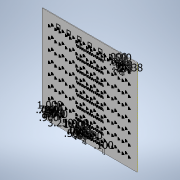
# Autodesk Inventor part: Cube_Pcb
Saved by Autodesk Inventor 2020 (Build 240168000, 168)
## iProperties
Created: 2019-12-01
Part Number: Cube_Pcb
Material: Generic
Document SubType Name: Modeling
Designer: torto
Density: 1 g/cm^3
Appearance: Default
Author: torto
Autodesk Inventor part; units mm, degrees
(part 1 of 2)
ref_plane "YZ Plane" through (0, 0, 0) normal (1, 0, 0) x (0, 1, 0)
ref_plane "XZ Plane" through (0, 0, 0) normal (0, 1, 0) x (-1, 0, 0)
ref_plane "XY Plane" through (0, 0, 0) normal (0, 0, 1) x (1, 0, 0)
sketch "Sketch1" plane through (0, 0, 0) normal (0, 0, 1) x (1, 0, 0)
  line L0 (0, 0) -> (228.6, 0)
  line L1 (228.6, 0) -> (228.6, 228.6)
  line L2 (228.6, 228.6) -> (0, 228.6)
  line L3 (0, 228.6) -> (0, 0)
  dimension "d0" = 228.6
  dimension "d1" = 228.6
  constraints: 8 end point, 2 parallel, 1 horizontal, 1 perpendicular
  measures "d0" distance of L2.end L1.end
  measures "d1" distance of L1.end L0.end
extrude "Extrusion1" add sketch "Sketch1" along normal blind 1.524
sketch "Details" plane through (0, 0, 1.524) normal (0, 0, 1) x (1, 0, 0)
  line L0 (0, 0) -> (82.55, 0) construction
  line L1 (82.55, 0) -> (82.55, 12.7) construction
  line L2 (82.55, 12.7) -> (0, 12.7) construction
  line L3 (0, 12.7) -> (0, 0) construction
  line L4 (82.55, 12.7) -> (146.05, 12.7)
  line L5 (146.05, 12.7) -> (146.05, 15.24)
  line L6 (146.05, 15.24) -> (82.55, 15.24)
  line L7 (82.55, 15.24) -> (82.55, 12.7)
  line L8 (82.55, 12.7) -> (100.33, 12.7)
  line L9 (100.33, 12.7) -> (100.33, 15.24)
  line L10 (100.33, 15.24) -> (82.55, 15.24)
  line L11 (82.55, 15.24) -> (82.55, 12.7)
  line L12 (105.41, 15.24) -> (105.41, 12.7)
  line L13 (123.19, 12.7) -> (123.19, 15.24)
  line L14 (128.27, 15.24) -> (128.27, 12.7)
  line L15 (146.05, 12.7) -> (146.05, 15.24)
  line L16 (82.55, 40.64) -> (82.55, 38.1)
  line L17 (82.55, 38.1) -> (100.33, 38.1)
  line L18 (100.33, 38.1) -> (100.33, 40.64)
  line L19 (100.33, 40.64) -> (82.55, 40.64)
  line L20 (146.05, 40.64) -> (82.55, 40.64)
  line L21 (105.41, 40.64) -> (105.41, 38.1)
  line L22 (82.55, 38.1) -> (146.05, 38.1)
  line L23 (146.05, 38.1) -> (146.05, 40.64)
  line L24 (128.27, 40.64) -> (128.27, 38.1)
  line L25 (123.19, 38.1) -> (123.19, 40.64)
  line L26 (82.55, 66.04) -> (82.55, 63.5)
  line L27 (82.55, 63.5) -> (100.33, 63.5)
  line L28 (100.33, 63.5) -> (100.33, 66.04)
  line L29 (100.33, 66.04) -> (82.55, 66.04)
  line L30 (146.05, 66.04) -> (82.55, 66.04)
  line L31 (105.41, 66.04) -> (105.41, 63.5)
  line L32 (82.55, 63.5) -> (146.05, 63.5)
  line L33 (146.05, 63.5) -> (146.05, 66.04)
  line L34 (128.27, 66.04) -> (128.27, 63.5)
  line L35 (123.19, 63.5) -> (123.19, 66.04)
  line L36 (82.55, 91.44) -> (82.55, 88.9)
  line L37 (82.55, 88.9) -> (100.33, 88.9)
  line L38 (100.33, 88.9) -> (100.33, 91.44)
  line L39 (100.33, 91.44) -> (82.55, 91.44)
  line L40 (146.05, 91.44) -> (82.55, 91.44)
  line L41 (105.41, 91.44) -> (105.41, 88.9)
  line L42 (82.55, 88.9) -> (146.05, 88.9)
  line L43 (146.05, 88.9) -> (146.05, 91.44)
  line L44 (128.27, 91.44) -> (128.27, 88.9)
  line L45 (123.19, 88.9) -> (123.19, 91.44)
  line L46 (82.55, 116.84) -> (82.55, 114.3)
  line L47 (82.55, 114.3) -> (100.33, 114.3)
  line L48 (100.33, 114.3) -> (100.33, 116.84)
  line L49 (100.33, 116.84) -> (82.55, 116.84)
  line L50 (146.05, 116.84) -> (82.55, 116.84)
  line L51 (105.41, 116.84) -> (105.41, 114.3)
  line L52 (82.55, 114.3) -> (146.05, 114.3)
  line L53 (146.05, 114.3) -> (146.05, 116.84)
  line L54 (128.27, 116.84) -> (128.27, 114.3)
  line L55 (123.19, 114.3) -> (123.19, 116.84)
  line L56 (82.55, 142.24) -> (82.55, 139.7)
  line L57 (82.55, 139.7) -> (100.33, 139.7)
  line L58 (100.33, 139.7) -> (100.33, 142.24)
  line L59 (100.33, 142.24) -> (82.55, 142.24)
  line L60 (146.05, 142.24) -> (82.55, 142.24)
  line L61 (105.41, 142.24) -> (105.41, 139.7)
  line L62 (82.55, 139.7) -> (146.05, 139.7)
  line L63 (146.05, 139.7) -> (146.05, 142.24)
  line L64 (128.27, 142.24) -> (128.27, 139.7)
  line L65 (123.19, 139.7) -> (123.19, 142.24)
  line L66 (82.55, 167.64) -> (82.55, 165.1)
  line L67 (82.55, 165.1) -> (100.33, 165.1)
  line L68 (100.33, 165.1) -> (100.33, 167.64)
  line L69 (100.33, 167.64) -> (82.55, 167.64)
  line L70 (146.05, 167.64) -> (82.55, 167.64)
  line L71 (105.41, 167.64) -> (105.41, 165.1)
  line L72 (82.55, 165.1) -> (146.05, 165.1)
  line L73 (146.05, 165.1) -> (146.05, 167.64)
  line L74 (128.27, 167.64) -> (128.27, 165.1)
  line L75 (123.19, 165.1) -> (123.19, 167.64)
  line L76 (82.55, 193.04) -> (82.55, 190.5)
  line L77 (82.55, 190.5) -> (100.33, 190.5)
  line L78 (100.33, 190.5) -> (100.33, 193.04)
  line L79 (100.33, 193.04) -> (82.55, 193.04)
  line L80 (146.05, 193.04) -> (82.55, 193.04)
  line L81 (105.41, 193.04) -> (105.41, 190.5)
  line L82 (82.55, 190.5) -> (146.05, 190.5)
  line L83 (146.05, 190.5) -> (146.05, 193.04)
  line L84 (128.27, 193.04) -> (128.27, 190.5)
  line L85 (123.19, 190.5) -> (123.19, 193.04)
  line L86 (82.55, 15.24) -> (83.185, 15.24) construction
  line L87 (83.185, 15.24) -> (83.185, 14.478) construction
  line L88 (83.185, 14.478) -> (82.55, 14.478) construction
  line L89 (82.55, 14.478) -> (82.55, 15.24) construction
  line L90 (83.185, 14.478) -> (81.915, 14.478)
  line L91 (81.915, 14.478) -> (81.915, 16.764)
  line L92 (81.915, 16.764) -> (83.185, 16.764)
  line L93 (83.185, 16.764) -> (83.185, 14.478)
  line L94 (86.995, 14.478) -> (86.995, 16.764)
  line L95 (86.995, 16.764) -> (88.265, 16.764)
  line L96 (88.265, 16.764) -> (88.265, 14.478)
  line L97 (88.265, 14.478) -> (86.995, 14.478)
  line L98 (92.075, 14.478) -> (92.075, 16.764)
  line L99 (92.075, 16.764) -> (93.345, 16.764)
  line L100 (93.345, 16.764) -> (93.345, 14.478)
  line L101 (93.345, 14.478) -> (92.075, 14.478)
  line L102 (97.155, 14.478) -> (97.155, 16.764)
  line L103 (97.155, 16.764) -> (98.425, 16.764)
  line L104 (98.425, 16.764) -> (98.425, 14.478)
  line L105 (98.425, 14.478) -> (97.155, 14.478)
  line L106 (100.33, 12.7) -> (99.695, 12.7) construction
  line L107 (99.695, 12.7) -> (99.695, 13.462) construction
  line L108 (99.695, 13.462) -> (100.33, 13.462) construction
  line L109 (100.33, 13.462) -> (100.33, 12.7) construction
  line L110 (99.695, 13.462) -> (100.9573, 13.462)
  line L111 (100.9573, 13.462) -> (100.9573, 11.176)
  line L112 (100.9573, 11.176) -> (99.695, 11.176)
  line L113 (99.695, 11.176) -> (99.695, 13.462)
  line L114 (94.615, 13.462) -> (95.8773, 13.462)
  line L115 (95.8773, 13.462) -> (95.8773, 11.176)
  line L116 (95.8773, 11.176) -> (94.615, 11.176)
  line L117 (94.615, 11.176) -> (94.615, 13.462)
  line L118 (89.535, 13.462) -> (90.7973, 13.462)
  line L119 (90.7973, 13.462) -> (90.7973, 11.176)
  line L120 (90.7973, 11.176) -> (89.535, 11.176)
  line L121 (89.535, 11.176) -> (89.535, 13.462)
  line L122 (84.455, 13.462) -> (85.7173, 13.462)
  line L123 (85.7173, 13.462) -> (85.7173, 11.176)
  line L124 (85.7173, 11.176) -> (84.455, 11.176)
  line L125 (84.455, 11.176) -> (84.455, 13.462)
  line L126 (81.915, 39.878) -> (81.915, 42.164)
  line L127 (81.915, 42.164) -> (83.185, 42.164)
  line L128 (83.185, 42.164) -> (83.185, 39.878)
  line L129 (83.185, 39.878) -> (81.915, 39.878)
  line L130 (84.455, 38.862) -> (85.7173, 38.862)
  line L131 (85.7173, 38.862) -> (85.7173, 36.576)
  line L132 (85.7173, 36.576) -> (84.455, 36.576)
  line L133 (84.455, 36.576) -> (84.455, 38.862)
  line L134 (88.265, 39.878) -> (86.995, 39.878)
  line L135 (88.265, 42.164) -> (88.265, 39.878)
  line L136 (86.995, 39.878) -> (86.995, 42.164)
  line L137 (86.995, 42.164) -> (88.265, 42.164)
  line L138 (89.535, 36.576) -> (89.535, 38.862)
  line L139 (90.7973, 36.576) -> (89.535, 36.576)
  line L140 (90.7973, 38.862) -> (90.7973, 36.576)
  line L141 (89.535, 38.862) -> (90.7973, 38.862)
  line L142 (92.075, 39.878) -> (92.075, 42.164)
  line L143 (93.345, 39.878) -> (92.075, 39.878)
  line L144 (93.345, 42.164) -> (93.345, 39.878)
  line L145 (92.075, 42.164) -> (93.345, 42.164)
  line L146 (94.615, 36.576) -> (94.615, 38.862)
  line L147 (94.615, 38.862) -> (95.8773, 38.862)
  line L148 (95.8773, 38.862) -> (95.8773, 36.576)
  line L149 (95.8773, 36.576) -> (94.615, 36.576)
  line L150 (97.155, 39.878) -> (97.155, 42.164)
  line L151 (97.155, 42.164) -> (98.425, 42.164)
  line L152 (98.425, 42.164) -> (98.425, 39.878)
  line L153 (98.425, 39.878) -> (97.155, 39.878)
  line L154 (99.695, 38.862) -> (100.9573, 38.862)
  line L155 (100.9573, 38.862) -> (100.9573, 36.576)
  line L156 (100.9573, 36.576) -> (99.695, 36.576)
  line L157 (99.695, 36.576) -> (99.695, 38.862)
  line L158 (81.915, 65.278) -> (81.915, 67.564)
  line L159 (81.915, 67.564) -> (83.185, 67.564)
  line L160 (83.185, 67.564) -> (83.185, 65.278)
  line L161 (83.185, 65.278) -> (81.915, 65.278)
  line L162 (84.455, 64.262) -> (85.7173, 64.262)
  line L163 (85.7173, 64.262) -> (85.7173, 61.976)
  line L164 (85.7173, 61.976) -> (84.455, 61.976)
  line L165 (84.455, 61.976) -> (84.455, 64.262)
  line L166 (88.265, 65.278) -> (86.995, 65.278)
  line L167 (88.265, 67.564) -> (88.265, 65.278)
  line L168 (86.995, 65.278) -> (86.995, 67.564)
  line L169 (86.995, 67.564) -> (88.265, 67.564)
  line L170 (89.535, 61.976) -> (89.535, 64.262)
  line L171 (90.7973, 61.976) -> (89.535, 61.976)
  line L172 (90.7973, 64.262) -> (90.7973, 61.976)
  line L173 (89.535, 64.262) -> (90.7973, 64.262)
  line L174 (92.075, 65.278) -> (92.075, 67.564)
  line L175 (93.345, 65.278) -> (92.075, 65.278)
  line L176 (93.345, 67.564) -> (93.345, 65.278)
  line L177 (92.075, 67.564) -> (93.345, 67.564)
  line L178 (94.615, 61.976) -> (94.615, 64.262)
  line L179 (94.615, 64.262) -> (95.8773, 64.262)
  line L180 (95.8773, 64.262) -> (95.8773, 61.976)
  line L181 (95.8773, 61.976) -> (94.615, 61.976)
  line L182 (97.155, 65.278) -> (97.155, 67.564)
  line L183 (97.155, 67.564) -> (98.425, 67.564)
  line L184 (98.425, 67.564) -> (98.425, 65.278)
  line L185 (98.425, 65.278) -> (97.155, 65.278)
  line L186 (99.695, 64.262) -> (100.9573, 64.262)
  line L187 (100.9573, 64.262) -> (100.9573, 61.976)
  line L188 (100.9573, 61.976) -> (99.695, 61.976)
  line L189 (99.695, 61.976) -> (99.695, 64.262)
  line L190 (81.915, 90.678) -> (81.915, 92.964)
  line L191 (81.915, 92.964) -> (83.185, 92.964)
  line L192 (83.185, 92.964) -> (83.185, 90.678)
  line L193 (83.185, 90.678) -> (81.915, 90.678)
  line L194 (84.455, 89.662) -> (85.7173, 89.662)
  line L195 (85.7173, 89.662) -> (85.7173, 87.376)
  line L196 (85.7173, 87.376) -> (84.455, 87.376)
  line L197 (84.455, 87.376) -> (84.455, 89.662)
  line L198 (88.265, 90.678) -> (86.995, 90.678)
  line L199 (88.265, 92.964) -> (88.265, 90.678)
  line L200 (86.995, 90.678) -> (86.995, 92.964)
  line L201 (86.995, 92.964) -> (88.265, 92.964)
  line L202 (89.535, 87.376) -> (89.535, 89.662)
  line L203 (90.7973, 87.376) -> (89.535, 87.376)
  line L204 (90.7973, 89.662) -> (90.7973, 87.376)
  line L205 (89.535, 89.662) -> (90.7973, 89.662)
  line L206 (92.075, 90.678) -> (92.075, 92.964)
  line L207 (93.345, 90.678) -> (92.075, 90.678)
  line L208 (93.345, 92.964) -> (93.345, 90.678)
  line L209 (92.075, 92.964) -> (93.345, 92.964)
  line L210 (94.615, 87.376) -> (94.615, 89.662)
  line L211 (94.615, 89.662) -> (95.8773, 89.662)
  line L212 (95.8773, 89.662) -> (95.8773, 87.376)
  line L213 (95.8773, 87.376) -> (94.615, 87.376)
  line L214 (97.155, 90.678) -> (97.155, 92.964)
  line L215 (97.155, 92.964) -> (98.425, 92.964)
  line L216 (98.425, 92.964) -> (98.425, 90.678)
  line L217 (98.425, 90.678) -> (97.155, 90.678)
  line L218 (99.695, 89.662) -> (100.9573, 89.662)
  line L219 (100.9573, 89.662) -> (100.9573, 87.376)
  line L220 (100.9573, 87.376) -> (99.695, 87.376)
  line L221 (99.695, 87.376) -> (99.695, 89.662)
  line L222 (81.915, 116.078) -> (81.915, 118.364)
  line L223 (81.915, 118.364) -> (83.185, 118.364)
  line L224 (83.185, 118.364) -> (83.185, 116.078)
  line L225 (83.185, 116.078) -> (81.915, 116.078)
  line L226 (84.455, 115.062) -> (85.7173, 115.062)
  line L227 (85.7173, 115.062) -> (85.7173, 112.776)
  line L228 (85.7173, 112.776) -> (84.455, 112.776)
  line L229 (84.455, 112.776) -> (84.455, 115.062)
  line L230 (88.265, 116.078) -> (86.995, 116.078)
  line L231 (88.265, 118.364) -> (88.265, 116.078)
  line L232 (86.995, 116.078) -> (86.995, 118.364)
  line L233 (86.995, 118.364) -> (88.265, 118.364)
  line L234 (89.535, 112.776) -> (89.535, 115.062)
  line L235 (90.7973, 112.776) -> (89.535, 112.776)
  line L236 (90.7973, 115.062) -> (90.7973, 112.776)
  line L237 (89.535, 115.062) -> (90.7973, 115.062)
  line L238 (92.075, 116.078) -> (92.075, 118.364)
  line L239 (93.345, 116.078) -> (92.075, 116.078)
  line L240 (93.345, 118.364) -> (93.345, 116.078)
  line L241 (92.075, 118.364) -> (93.345, 118.364)
  line L242 (94.615, 112.776) -> (94.615, 115.062)
  line L243 (94.615, 115.062) -> (95.8773, 115.062)
  line L244 (95.8773, 115.062) -> (95.8773, 112.776)
  line L245 (95.8773, 112.776) -> (94.615, 112.776)
  line L246 (97.155, 116.078) -> (97.155, 118.364)
  line L247 (97.155, 118.364) -> (98.425, 118.364)
  line L248 (98.425, 118.364) -> (98.425, 116.078)
  line L249 (98.425, 116.078) -> (97.155, 116.078)
  line L250 (99.695, 115.062) -> (100.9573, 115.062)
  line L251 (100.9573, 115.062) -> (100.9573, 112.776)
  line L252 (100.9573, 112.776) -> (99.695, 112.776)
  line L253 (99.695, 112.776) -> (99.695, 115.062)
  line L254 (81.915, 141.478) -> (81.915, 143.764)
  line L255 (81.915, 143.764) -> (83.185, 143.764)
  line L256 (83.185, 143.764) -> (83.185, 141.478)
  line L257 (83.185, 141.478) -> (81.915, 141.478)
  line L258 (84.455, 140.462) -> (85.7173, 140.462)
  line L259 (85.7173, 140.462) -> (85.7173, 138.176)
  line L260 (85.7173, 138.176) -> (84.455, 138.176)
  line L261 (84.455, 138.176) -> (84.455, 140.462)
  line L262 (88.265, 141.478) -> (86.995, 141.478)
  line L263 (88.265, 143.764) -> (88.265, 141.478)
  line L264 (86.995, 141.478) -> (86.995, 143.764)
  line L265 (86.995, 143.764) -> (88.265, 143.764)
  line L266 (89.535, 138.176) -> (89.535, 140.462)
  line L267 (90.7973, 138.176) -> (89.535, 138.176)
  line L268 (90.7973, 140.462) -> (90.7973, 138.176)
  line L269 (89.535, 140.462) -> (90.7973, 140.462)
  line L270 (92.075, 141.478) -> (92.075, 143.764)
  line L271 (93.345, 141.478) -> (92.075, 141.478)
  line L272 (93.345, 143.764) -> (93.345, 141.478)
  line L273 (92.075, 143.764) -> (93.345, 143.764)
  line L274 (94.615, 138.176) -> (94.615, 140.462)
  line L275 (94.615, 140.462) -> (95.8773, 140.462)
  line L276 (95.8773, 140.462) -> (95.8773, 138.176)
  line L277 (95.8773, 138.176) -> (94.615, 138.176)
  line L278 (97.155, 141.478) -> (97.155, 143.764)
  line L279 (97.155, 143.764) -> (98.425, 143.764)
  line L280 (98.425, 143.764) -> (98.425, 141.478)
  line L281 (98.425, 141.478) -> (97.155, 141.478)
  line L282 (99.695, 140.462) -> (100.9573, 140.462)
  line L283 (100.9573, 140.462) -> (100.9573, 138.176)
  line L284 (100.9573, 138.176) -> (99.695, 138.176)
  line L285 (99.695, 138.176) -> (99.695, 140.462)
  line L286 (81.915, 166.878) -> (81.915, 169.164)
  line L287 (81.915, 169.164) -> (83.185, 169.164)
  line L288 (83.185, 169.164) -> (83.185, 166.878)
  line L289 (83.185, 166.878) -> (81.915, 166.878)
  line L290 (84.455, 165.862) -> (85.7173, 165.862)
  line L291 (85.7173, 165.862) -> (85.7173, 163.576)
  line L292 (85.7173, 163.576) -> (84.455, 163.576)
  line L293 (84.455, 163.576) -> (84.455, 165.862)
  line L294 (88.265, 166.878) -> (86.995, 166.878)
  line L295 (88.265, 169.164) -> (88.265, 166.878)
  line L296 (86.995, 166.878) -> (86.995, 169.164)
  line L297 (86.995, 169.164) -> (88.265, 169.164)
  line L298 (89.535, 163.576) -> (89.535, 165.862)
  line L299 (90.7973, 163.576) -> (89.535, 163.576)
  line L300 (90.7973, 165.862) -> (90.7973, 163.576)
  line L301 (89.535, 165.862) -> (90.7973, 165.862)
  line L302 (92.075, 166.878) -> (92.075, 169.164)
  line L303 (93.345, 166.878) -> (92.075, 166.878)
  line L304 (93.345, 169.164) -> (93.345, 166.878)
  line L305 (92.075, 169.164) -> (93.345, 169.164)
  line L306 (94.615, 163.576) -> (94.615, 165.862)
  line L307 (94.615, 165.862) -> (95.8773, 165.862)
  line L308 (95.8773, 165.862) -> (95.8773, 163.576)
  line L309 (95.8773, 163.576) -> (94.615, 163.576)
  line L310 (97.155, 166.878) -> (97.155, 169.164)
  line L311 (97.155, 169.164) -> (98.425, 169.164)
  line L312 (98.425, 169.164) -> (98.425, 166.878)
  line L313 (98.425, 166.878) -> (97.155, 166.878)
  line L314 (99.695, 165.862) -> (100.9573, 165.862)
  line L315 (100.9573, 165.862) -> (100.9573, 163.576)
  line L316 (100.9573, 163.576) -> (99.695, 163.576)
  line L317 (99.695, 163.576) -> (99.695, 165.862)
  line L318 (81.915, 192.278) -> (81.915, 194.564)
  line L319 (81.915, 194.564) -> (83.185, 194.564)
  line L320 (83.185, 194.564) -> (83.185, 192.278)
  line L321 (83.185, 192.278) -> (81.915, 192.278)
  line L322 (84.455, 191.262) -> (85.7173, 191.262)
  line L323 (85.7173, 191.262) -> (85.7173, 188.976)
  line L324 (85.7173, 188.976) -> (84.455, 188.976)
  line L325 (84.455, 188.976) -> (84.455, 191.262)
  line L326 (88.265, 192.278) -> (86.995, 192.278)
  line L327 (88.265, 194.564) -> (88.265, 192.278)
  line L328 (86.995, 192.278) -> (86.995, 194.564)
  line L329 (86.995, 194.564) -> (88.265, 194.564)
  line L330 (89.535, 188.976) -> (89.535, 191.262)
  line L331 (90.7973, 188.976) -> (89.535, 188.976)
  line L332 (90.7973, 191.262) -> (90.7973, 188.976)
  line L333 (89.535, 191.262) -> (90.7973, 191.262)
  line L334 (92.075, 192.278) -> (92.075, 194.564)
  line L335 (93.345, 192.278) -> (92.075, 192.278)
  line L336 (93.345, 194.564) -> (93.345, 192.278)
  line L337 (92.075, 194.564) -> (93.345, 194.564)
  line L338 (94.615, 188.976) -> (94.615, 191.262)
  line L339 (94.615, 191.262) -> (95.8773, 191.262)
  line L340 (95.8773, 191.262) -> (95.8773, 188.976)
  line L341 (95.8773, 188.976) -> (94.615, 188.976)
  line L342 (97.155, 192.278) -> (97.155, 194.564)
  line L343 (97.155, 194.564) -> (98.425, 194.564)
  line L344 (98.425, 194.564) -> (98.425, 192.278)
  line L345 (98.425, 192.278) -> (97.155, 192.278)
  line L346 (99.695, 191.262) -> (100.9573, 191.262)
  line L347 (100.9573, 191.262) -> (100.9573, 188.976)
  line L348 (100.9573, 188.976) -> (99.695, 188.976)
  line L349 (99.695, 188.976) -> (99.695, 191.262)
  line L350 (104.775, 14.478) -> (104.775, 16.764)
  line L351 (104.775, 16.764) -> (106.045, 16.764)
  line L352 (106.045, 16.764) -> (106.045, 14.478)
  line L353 (106.045, 14.478) -> (104.775, 14.478)
  line L354 (107.315, 13.462) -> (108.5773, 13.462)
  line L355 (108.5773, 13.462) -> (108.5773, 11.176)
  line L356 (108.5773, 11.176) -> (107.315, 11.176)
  line L357 (107.315, 11.176) -> (107.315, 13.462)
  line L358 (111.125, 14.478) -> (109.855, 14.478)
  line L359 (111.125, 16.764) -> (111.125, 14.478)
  line L360 (109.855, 14.478) -> (109.855, 16.764)
  line L361 (109.855, 16.764) -> (111.125, 16.764)
  line L362 (112.395, 11.176) -> (112.395, 13.462)
  line L363 (113.6573, 11.176) -> (112.395, 11.176)
  line L364 (113.6573, 13.462) -> (113.6573, 11.176)
  line L365 (112.395, 13.462) -> (113.6573, 13.462)
  line L366 (114.935, 14.478) -> (114.935, 16.764)
  line L367 (116.205, 14.478) -> (114.935, 14.478)
  line L368 (116.205, 16.764) -> (116.205, 14.478)
  line L369 (114.935, 16.764) -> (116.205, 16.764)
  line L370 (117.475, 11.176) -> (117.475, 13.462)
  line L371 (117.475, 13.462) -> (118.7373, 13.462)
  line L372 (118.7373, 13.462) -> (118.7373, 11.176)
  line L373 (118.7373, 11.176) -> (117.475, 11.176)
  line L374 (120.015, 14.478) -> (120.015, 16.764)
  line L375 (120.015, 16.764) -> (121.285, 16.764)
  line L376 (121.285, 16.764) -> (121.285, 14.478)
  line L377 (121.285, 14.478) -> (120.015, 14.478)
  line L378 (122.555, 13.462) -> (123.8173, 13.462)
  line L379 (123.8173, 13.462) -> (123.8173, 11.176)
  line L380 (123.8173, 11.176) -> (122.555, 11.176)
  line L381 (122.555, 11.176) -> (122.555, 13.462)
  line L382 (104.775, 39.878) -> (104.775, 42.164)
  line L383 (104.775, 42.164) -> (106.045, 42.164)
  line L384 (106.045, 42.164) -> (106.045, 39.878)
  line L385 (106.045, 39.878) -> (104.775, 39.878)
  line L386 (107.315, 38.862) -> (108.5773, 38.862)
  line L387 (108.5773, 38.862) -> (108.5773, 36.576)
  line L388 (108.5773, 36.576) -> (107.315, 36.576)
  line L389 (107.315, 36.576) -> (107.315, 38.862)
  line L390 (111.125, 39.878) -> (109.855, 39.878)
  line L391 (111.125, 42.164) -> (111.125, 39.878)
  line L392 (109.855, 39.878) -> (109.855, 42.164)
  line L393 (109.855, 42.164) -> (111.125, 42.164)
  line L394 (112.395, 36.576) -> (112.395, 38.862)
  line L395 (113.6573, 36.576) -> (112.395, 36.576)
  line L396 (113.6573, 38.862) -> (113.6573, 36.576)
  line L397 (112.395, 38.862) -> (113.6573, 38.862)
  line L398 (114.935, 39.878) -> (114.935, 42.164)
  line L399 (116.205, 39.878) -> (114.935, 39.878)
  line L400 (116.205, 42.164) -> (116.205, 39.878)
  line L401 (114.935, 42.164) -> (116.205, 42.164)
  line L402 (117.475, 36.576) -> (117.475, 38.862)
  line L403 (117.475, 38.862) -> (118.7373, 38.862)
  line L404 (118.7373, 38.862) -> (118.7373, 36.576)
  line L405 (118.7373, 36.576) -> (117.475, 36.576)
  line L406 (120.015, 39.878) -> (120.015, 42.164)
  line L407 (120.015, 42.164) -> (121.285, 42.164)
  line L408 (121.285, 42.164) -> (121.285, 39.878)
  line L409 (121.285, 39.878) -> (120.015, 39.878)
  line L410 (122.555, 38.862) -> (123.8173, 38.862)
  line L411 (123.8173, 38.862) -> (123.8173, 36.576)
  line L412 (123.8173, 36.576) -> (122.555, 36.576)
  line L413 (122.555, 36.576) -> (122.555, 38.862)
  line L414 (104.775, 65.278) -> (104.775, 67.564)
  line L415 (104.775, 67.564) -> (106.045, 67.564)
  line L416 (106.045, 67.564) -> (106.045, 65.278)
  line L417 (106.045, 65.278) -> (104.775, 65.278)
  line L418 (107.315, 64.262) -> (108.5773, 64.262)
  line L419 (108.5773, 64.262) -> (108.5773, 61.976)
  line L420 (108.5773, 61.976) -> (107.315, 61.976)
  line L421 (107.315, 61.976) -> (107.315, 64.262)
  line L422 (111.125, 65.278) -> (109.855, 65.278)
  line L423 (111.125, 67.564) -> (111.125, 65.278)
  line L424 (109.855, 65.278) -> (109.855, 67.564)
  line L425 (109.855, 67.564) -> (111.125, 67.564)
  line L426 (112.395, 61.976) -> (112.395, 64.262)
  line L427 (113.6573, 61.976) -> (112.395, 61.976)
  line L428 (113.6573, 64.262) -> (113.6573, 61.976)
  line L429 (112.395, 64.262) -> (113.6573, 64.262)
  line L430 (114.935, 65.278) -> (114.935, 67.564)
  line L431 (116.205, 65.278) -> (114.935, 65.278)
  line L432 (116.205, 67.564) -> (116.205, 65.278)
  line L433 (114.935, 67.564) -> (116.205, 67.564)
  line L434 (117.475, 61.976) -> (117.475, 64.262)
  line L435 (117.475, 64.262) -> (118.7373, 64.262)
  line L436 (118.7373, 64.262) -> (118.7373, 61.976)
  line L437 (118.7373, 61.976) -> (117.475, 61.976)
  line L438 (120.015, 65.278) -> (120.015, 67.564)
  line L439 (120.015, 67.564) -> (121.285, 67.564)
  line L440 (121.285, 67.564) -> (121.285, 65.278)
  line L441 (121.285, 65.278) -> (120.015, 65.278)
  line L442 (122.555, 64.262) -> (123.8173, 64.262)
  line L443 (123.8173, 64.262) -> (123.8173, 61.976)
  line L444 (123.8173, 61.976) -> (122.555, 61.976)
  line L445 (122.555, 61.976) -> (122.555, 64.262)
  line L446 (104.775, 90.678) -> (104.775, 92.964)
  line L447 (104.775, 92.964) -> (106.045, 92.964)
  line L448 (106.045, 92.964) -> (106.045, 90.678)
  line L449 (106.045, 90.678) -> (104.775, 90.678)
  line L450 (107.315, 89.662) -> (108.5773, 89.662)
  line L451 (108.5773, 89.662) -> (108.5773, 87.376)
  line L452 (108.5773, 87.376) -> (107.315, 87.376)
  line L453 (107.315, 87.376) -> (107.315, 89.662)
  line L454 (111.125, 90.678) -> (109.855, 90.678)
  line L455 (111.125, 92.964) -> (111.125, 90.678)
  line L456 (109.855, 90.678) -> (109.855, 92.964)
  line L457 (109.855, 92.964) -> (111.125, 92.964)
  line L458 (112.395, 87.376) -> (112.395, 89.662)
  line L459 (113.6573, 87.376) -> (112.395, 87.376)
  line L460 (113.6573, 89.662) -> (113.6573, 87.376)
  line L461 (112.395, 89.662) -> (113.6573, 89.662)
  line L462 (114.935, 90.678) -> (114.935, 92.964)
  line L463 (116.205, 90.678) -> (114.935, 90.678)
  line L464 (116.205, 92.964) -> (116.205, 90.678)
  line L465 (114.935, 92.964) -> (116.205, 92.964)
  line L466 (117.475, 87.376) -> (117.475, 89.662)
  line L467 (117.475, 89.662) -> (118.7373, 89.662)
  line L468 (118.7373, 89.662) -> (118.7373, 87.376)
  line L469 (118.7373, 87.376) -> (117.475, 87.376)
  line L470 (120.015, 90.678) -> (120.015, 92.964)
  line L471 (120.015, 92.964) -> (121.285, 92.964)
  line L472 (121.285, 92.964) -> (121.285, 90.678)
  line L473 (121.285, 90.678) -> (120.015, 90.678)
  line L474 (122.555, 89.662) -> (123.8173, 89.662)
  line L475 (123.8173, 89.662) -> (123.8173, 87.376)
  line L476 (123.8173, 87.376) -> (122.555, 87.376)
  line L477 (122.555, 87.376) -> (122.555, 89.662)
  line L478 (104.775, 116.078) -> (104.775, 118.364)
  line L479 (104.775, 118.364) -> (106.045, 118.364)
  line L480 (106.045, 118.364) -> (106.045, 116.078)
  line L481 (106.045, 116.078) -> (104.775, 116.078)
  line L482 (107.315, 115.062) -> (108.5773, 115.062)
  line L483 (108.5773, 115.062) -> (108.5773, 112.776)
  line L484 (108.5773, 112.776) -> (107.315, 112.776)
  line L485 (107.315, 112.776) -> (107.315, 115.062)
  line L486 (111.125, 116.078) -> (109.855, 116.078)
  line L487 (111.125, 118.364) -> (111.125, 116.078)
  line L488 (109.855, 116.078) -> (109.855, 118.364)
  line L489 (109.855, 118.364) -> (111.125, 118.364)
  line L490 (112.395, 112.776) -> (112.395, 115.062)
  line L491 (113.6573, 112.776) -> (112.395, 112.776)
  line L492 (113.6573, 115.062) -> (113.6573, 112.776)
  line L493 (112.395, 115.062) -> (113.6573, 115.062)
  line L494 (114.935, 116.078) -> (114.935, 118.364)
  line L495 (116.205, 116.078) -> (114.935, 116.078)
  line L496 (116.205, 118.364) -> (116.205, 116.078)
  line L497 (114.935, 118.364) -> (116.205, 118.364)
  line L498 (117.475, 112.776) -> (117.475, 115.062)
  line L499 (117.475, 115.062) -> (118.7373, 115.062)
  line L500 (118.7373, 115.062) -> (118.7373, 112.776)
  line L501 (118.7373, 112.776) -> (117.475, 112.776)
  line L502 (120.015, 116.078) -> (120.015, 118.364)
  line L503 (120.015, 118.364) -> (121.285, 118.364)
  line L504 (121.285, 118.364) -> (121.285, 116.078)
  line L505 (121.285, 116.078) -> (120.015, 116.078)
  line L506 (122.555, 115.062) -> (123.8173, 115.062)
  line L507 (123.8173, 115.062) -> (123.8173, 112.776)
  line L508 (123.8173, 112.776) -> (122.555, 112.776)
  line L509 (122.555, 112.776) -> (122.555, 115.062)
  line L510 (104.775, 141.478) -> (104.775, 143.764)
  line L511 (104.775, 143.764) -> (106.045, 143.764)
  line L512 (106.045, 143.764) -> (106.045, 141.478)
  line L513 (106.045, 141.478) -> (104.775, 141.478)
  line L514 (107.315, 140.462) -> (108.5773, 140.462)
  line L515 (108.5773, 140.462) -> (108.5773, 138.176)
  line L516 (108.5773, 138.176) -> (107.315, 138.176)
  line L517 (107.315, 138.176) -> (107.315, 140.462)
  line L518 (111.125, 141.478) -> (109.855, 141.478)
  line L519 (111.125, 143.764) -> (111.125, 141.478)
  line L520 (109.855, 141.478) -> (109.855, 143.764)
  line L521 (109.855, 143.764) -> (111.125, 143.764)
  line L522 (112.395, 138.176) -> (112.395, 140.462)
  line L523 (113.6573, 138.176) -> (112.395, 138.176)
  line L524 (113.6573, 140.462) -> (113.6573, 138.176)
  line L525 (112.395, 140.462) -> (113.6573, 140.462)
  line L526 (114.935, 141.478) -> (114.935, 143.764)
  line L527 (116.205, 141.478) -> (114.935, 141.478)
  line L528 (116.205, 143.764) -> (116.205, 141.478)
  line L529 (114.935, 143.764) -> (116.205, 143.764)
  line L530 (117.475, 138.176) -> (117.475, 140.462)
  line L531 (117.475, 140.462) -> (118.7373, 140.462)
  line L532 (118.7373, 140.462) -> (118.7373, 138.176)
  line L533 (118.7373, 138.176) -> (117.475, 138.176)
  line L534 (120.015, 141.478) -> (120.015, 143.764)
  line L535 (120.015, 143.764) -> (121.285, 143.764)
  line L536 (121.285, 143.764) -> (121.285, 141.478)
  line L537 (121.285, 141.478) -> (120.015, 141.478)
  line L538 (122.555, 140.462) -> (123.8173, 140.462)
  line L539 (123.8173, 140.462) -> (123.8173, 138.176)
  line L540 (123.8173, 138.176) -> (122.555, 138.176)
  line L541 (122.555, 138.176) -> (122.555, 140.462)
  line L542 (104.775, 166.878) -> (104.775, 169.164)
  line L543 (104.775, 169.164) -> (106.045, 169.164)
  line L544 (106.045, 169.164) -> (106.045, 166.878)
  line L545 (106.045, 166.878) -> (104.775, 166.878)
  line L546 (107.315, 165.862) -> (108.5773, 165.862)
  line L547 (108.5773, 165.862) -> (108.5773, 163.576)
  line L548 (108.5773, 163.576) -> (107.315, 163.576)
  line L549 (107.315, 163.576) -> (107.315, 165.862)
  line L550 (111.125, 166.878) -> (109.855, 166.878)
  line L551 (111.125, 169.164) -> (111.125, 166.878)
  line L552 (109.855, 166.878) -> (109.855, 169.164)
  line L553 (109.855, 169.164) -> (111.125, 169.164)
  line L554 (112.395, 163.576) -> (112.395, 165.862)
  line L555 (113.6573, 163.576) -> (112.395, 163.576)
  line L556 (113.6573, 165.862) -> (113.6573, 163.576)
  line L557 (112.395, 165.862) -> (113.6573, 165.862)
  line L558 (114.935, 166.878) -> (114.935, 169.164)
  line L559 (116.205, 166.878) -> (114.935, 166.878)
  line L560 (116.205, 169.164) -> (116.205, 166.878)
  line L561 (114.935, 169.164) -> (116.205, 169.164)
  line L562 (117.475, 163.576) -> (117.475, 165.862)
  line L563 (117.475, 165.862) -> (118.7373, 165.862)
  line L564 (118.7373, 165.862) -> (118.7373, 163.576)
  line L565 (118.7373, 163.576) -> (117.475, 163.576)
  line L566 (120.015, 166.878) -> (120.015, 169.164)
  line L567 (120.015, 169.164) -> (121.285, 169.164)
  line L568 (121.285, 169.164) -> (121.285, 166.878)
  line L569 (121.285, 166.878) -> (120.015, 166.878)
  line L570 (122.555, 165.862) -> (123.8173, 165.862)
  line L571 (123.8173, 165.862) -> (123.8173, 163.576)
  line L572 (123.8173, 163.576) -> (122.555, 163.576)
  line L573 (122.555, 163.576) -> (122.555, 165.862)
  line L574 (104.775, 192.278) -> (104.775, 194.564)
  line L575 (104.775, 194.564) -> (106.045, 194.564)
  line L576 (106.045, 194.564) -> (106.045, 192.278)
  line L577 (106.045, 192.278) -> (104.775, 192.278)
  line L578 (107.315, 191.262) -> (108.5773, 191.262)
  line L579 (108.5773, 191.262) -> (108.5773, 188.976)
  line L580 (108.5773, 188.976) -> (107.315, 188.976)
  line L581 (107.315, 188.976) -> (107.315, 191.262)
  line L582 (111.125, 192.278) -> (109.855, 192.278)
  line L583 (111.125, 194.564) -> (111.125, 192.278)
  line L584 (109.855, 192.278) -> (109.855, 194.564)
  line L585 (109.855, 194.564) -> (111.125, 194.564)
  line L586 (112.395, 188.976) -> (112.395, 191.262)
  line L587 (113.6573, 188.976) -> (112.395, 188.976)
  line L588 (113.6573, 191.262) -> (113.6573, 188.976)
  line L589 (112.395, 191.262) -> (113.6573, 191.262)
  line L590 (114.935, 192.278) -> (114.935, 194.564)
  line L591 (116.205, 192.278) -> (114.935, 192.278)
  line L592 (116.205, 194.564) -> (116.205, 192.278)
  line L593 (114.935, 194.564) -> (116.205, 194.564)
  line L594 (117.475, 188.976) -> (117.475, 191.262)
  line L595 (117.475, 191.262) -> (118.7373, 191.262)
  line L596 (118.7373, 191.262) -> (118.7373, 188.976)
  line L597 (118.7373, 188.976) -> (117.475, 188.976)
  line L598 (120.015, 192.278) -> (120.015, 194.564)
  line L599 (120.015, 194.564) -> (121.285, 194.564)
  line L600 (121.285, 194.564) -> (121.285, 192.278)
  line L601 (121.285, 192.278) -> (120.015, 192.278)
  line L602 (122.555, 191.262) -> (123.8173, 191.262)
  line L603 (123.8173, 191.262) -> (123.8173, 188.976)
  line L604 (123.8173, 188.976) -> (122.555, 188.976)
  line L605 (122.555, 188.976) -> (122.555, 191.262)
  line L606 (127.635, 14.478) -> (127.635, 16.764)
  line L607 (127.635, 16.764) -> (128.905, 16.764)
  line L608 (128.905, 16.764) -> (128.905, 14.478)
  line L609 (128.905, 14.478) -> (127.635, 14.478)
  line L610 (130.175, 13.462) -> (131.4373, 13.462)
  line L611 (131.4373, 13.462) -> (131.4373, 11.176)
  line L612 (131.4373, 11.176) -> (130.175, 11.176)
  line L613 (130.175, 11.176) -> (130.175, 13.462)
  line L614 (133.985, 14.478) -> (132.715, 14.478)
  line L615 (133.985, 16.764) -> (133.985, 14.478)
  line L616 (132.715, 14.478) -> (132.715, 16.764)
  line L617 (132.715, 16.764) -> (133.985, 16.764)
  line L618 (135.255, 11.176) -> (135.255, 13.462)
  line L619 (136.5173, 11.176) -> (135.255, 11.176)
  line L620 (136.5173, 13.462) -> (136.5173, 11.176)
  line L621 (135.255, 13.462) -> (136.5173, 13.462)
  line L622 (137.795, 14.478) -> (137.795, 16.764)
  line L623 (139.065, 14.478) -> (137.795, 14.478)
  line L624 (139.065, 16.764) -> (139.065, 14.478)
  line L625 (137.795, 16.764) -> (139.065, 16.764)
  line L626 (140.335, 11.176) -> (140.335, 13.462)
  line L627 (140.335, 13.462) -> (141.5973, 13.462)
  line L628 (141.5973, 13.462) -> (141.5973, 11.176)
  line L629 (141.5973, 11.176) -> (140.335, 11.176)
  line L630 (142.875, 14.478) -> (142.875, 16.764)
  line L631 (142.875, 16.764) -> (144.145, 16.764)
  line L632 (144.145, 16.764) -> (144.145, 14.478)
  line L633 (144.145, 14.478) -> (142.875, 14.478)
  line L634 (145.415, 13.462) -> (146.6773, 13.462)
  line L635 (146.6773, 13.462) -> (146.6773, 11.176)
  line L636 (146.6773, 11.176) -> (145.415, 11.176)
  line L637 (145.415, 11.176) -> (145.415, 13.462)
  line L638 (127.635, 39.878) -> (127.635, 42.164)
  line L639 (127.635, 42.164) -> (128.905, 42.164)
  line L640 (128.905, 42.164) -> (128.905, 39.878)
  line L641 (128.905, 39.878) -> (127.635, 39.878)
  line L642 (130.175, 38.862) -> (131.4373, 38.862)
  line L643 (131.4373, 38.862) -> (131.4373, 36.576)
  line L644 (131.4373, 36.576) -> (130.175, 36.576)
  line L645 (130.175, 36.576) -> (130.175, 38.862)
  line L646 (133.985, 39.878) -> (132.715, 39.878)
  line L647 (133.985, 42.164) -> (133.985, 39.878)
  line L648 (132.715, 39.878) -> (132.715, 42.164)
  line L649 (132.715, 42.164) -> (133.985, 42.164)
  line L650 (135.255, 36.576) -> (135.255, 38.862)
  line L651 (136.5173, 36.576) -> (135.255, 36.576)
  line L652 (136.5173, 38.862) -> (136.5173, 36.576)
  line L653 (135.255, 38.862) -> (136.5173, 38.862)
  line L654 (137.795, 39.878) -> (137.795, 42.164)
  line L655 (139.065, 39.878) -> (137.795, 39.878)
  line L656 (139.065, 42.164) -> (139.065, 39.878)
  line L657 (137.795, 42.164) -> (139.065, 42.164)
  line L658 (140.335, 36.576) -> (140.335, 38.862)
  line L659 (140.335, 38.862) -> (141.5973, 38.862)
  line L660 (141.5973, 38.862) -> (141.5973, 36.576)
  line L661 (141.5973, 36.576) -> (140.335, 36.576)
  line L662 (142.875, 39.878) -> (142.875, 42.164)
  line L663 (142.875, 42.164) -> (144.145, 42.164)
  line L664 (144.145, 42.164) -> (144.145, 39.878)
  line L665 (144.145, 39.878) -> (142.875, 39.878)
  line L666 (145.415, 38.862) -> (146.6773, 38.862)
  line L667 (146.6773, 38.862) -> (146.6773, 36.576)
  line L668 (146.6773, 36.576) -> (145.415, 36.576)
  line L669 (145.415, 36.576) -> (145.415, 38.862)
  line L670 (127.635, 65.278) -> (127.635, 67.564)
  line L671 (127.635, 67.564) -> (128.905, 67.564)
  line L672 (128.905, 67.564) -> (128.905, 65.278)
  line L673 (128.905, 65.278) -> (127.635, 65.278)
  line L674 (130.175, 64.262) -> (131.4373, 64.262)
  line L675 (131.4373, 64.262) -> (131.4373, 61.976)
  line L676 (131.4373, 61.976) -> (130.175, 61.976)
  line L677 (130.175, 61.976) -> (130.175, 64.262)
  line L678 (133.985, 65.278) -> (132.715, 65.278)
  line L679 (133.985, 67.564) -> (133.985, 65.278)
  line L680 (132.715, 65.278) -> (132.715, 67.564)
  line L681 (132.715, 67.564) -> (133.985, 67.564)
  line L682 (135.255, 61.976) -> (135.255, 64.262)
  line L683 (136.5173, 61.976) -> (135.255, 61.976)
  line L684 (136.5173, 64.262) -> (136.5173, 61.976)
  line L685 (135.255, 64.262) -> (136.5173, 64.262)
  line L686 (137.795, 65.278) -> (137.795, 67.564)
  line L687 (139.065, 65.278) -> (137.795, 65.278)
  line L688 (139.065, 67.564) -> (139.065, 65.278)
  line L689 (137.795, 67.564) -> (139.065, 67.564)
  line L690 (140.335, 61.976) -> (140.335, 64.262)
  line L691 (140.335, 64.262) -> (141.5973, 64.262)
  line L692 (141.5973, 64.262) -> (141.5973, 61.976)
  line L693 (141.5973, 61.976) -> (140.335, 61.976)
  line L694 (142.875, 65.278) -> (142.875, 67.564)
  line L695 (142.875, 67.564) -> (144.145, 67.564)
  line L696 (144.145, 67.564) -> (144.145, 65.278)
  line L697 (144.145, 65.278) -> (142.875, 65.278)
  line L698 (145.415, 64.262) -> (146.6773, 64.262)
  line L699 (146.6773, 64.262) -> (146.6773, 61.976)
  line L700 (146.6773, 61.976) -> (145.415, 61.976)
  line L701 (145.415, 61.976) -> (145.415, 64.262)
  line L702 (127.635, 90.678) -> (127.635, 92.964)
  line L703 (127.635, 92.964) -> (128.905, 92.964)
  line L704 (128.905, 92.964) -> (128.905, 90.678)
  line L705 (128.905, 90.678) -> (127.635, 90.678)
  line L706 (130.175, 89.662) -> (131.4373, 89.662)
  line L707 (131.4373, 89.662) -> (131.4373, 87.376)
  line L708 (131.4373, 87.376) -> (130.175, 87.376)
  line L709 (130.175, 87.376) -> (130.175, 89.662)
  line L710 (133.985, 90.678) -> (132.715, 90.678)
  line L711 (133.985, 92.964) -> (133.985, 90.678)
  line L712 (132.715, 90.678) -> (132.715, 92.964)
  line L713 (132.715, 92.964) -> (133.985, 92.964)
  line L714 (135.255, 87.376) -> (135.255, 89.662)
  line L715 (136.5173, 87.376) -> (135.255, 87.376)
  line L716 (136.5173, 89.662) -> (136.5173, 87.376)
  line L717 (135.255, 89.662) -> (136.5173, 89.662)
  line L718 (137.795, 90.678) -> (137.795, 92.964)
  line L719 (139.065, 90.678) -> (137.795, 90.678)
  line L720 (139.065, 92.964) -> (139.065, 90.678)
  line L721 (137.795, 92.964) -> (139.065, 92.964)
  line L722 (140.335, 87.376) -> (140.335, 89.662)
  line L723 (140.335, 89.662) -> (141.5973, 89.662)
  line L724 (141.5973, 89.662) -> (141.5973, 87.376)
  line L725 (141.5973, 87.376) -> (140.335, 87.376)
  line L726 (142.875, 90.678) -> (142.875, 92.964)
  line L727 (142.875, 92.964) -> (144.145, 92.964)
  line L728 (144.145, 92.964) -> (144.145, 90.678)
  line L729 (144.145, 90.678) -> (142.875, 90.678)
  line L730 (145.415, 89.662) -> (146.6773, 89.662)
  line L731 (146.6773, 89.662) -> (146.6773, 87.376)
  line L732 (146.6773, 87.376) -> (145.415, 87.376)
  line L733 (145.415, 87.376) -> (145.415, 89.662)
  line L734 (127.635, 116.078) -> (127.635, 118.364)
  line L735 (127.635, 118.364) -> (128.905, 118.364)
  line L736 (128.905, 118.364) -> (128.905, 116.078)
  line L737 (128.905, 116.078) -> (127.635, 116.078)
  line L738 (130.175, 115.062) -> (131.4373, 115.062)
  line L739 (131.4373, 115.062) -> (131.4373, 112.776)
  line L740 (131.4373, 112.776) -> (130.175, 112.776)
  line L741 (130.175, 112.776) -> (130.175, 115.062)
  line L742 (133.985, 116.078) -> (132.715, 116.078)
  line L743 (133.985, 118.364) -> (133.985, 116.078)
  line L744 (132.715, 116.078) -> (132.715, 118.364)
  line L745 (132.715, 118.364) -> (133.985, 118.364)
  line L746 (135.255, 112.776) -> (135.255, 115.062)
  line L747 (136.5173, 112.776) -> (135.255, 112.776)
  line L748 (136.5173, 115.062) -> (136.5173, 112.776)
  line L749 (135.255, 115.062) -> (136.5173, 115.062)
  line L750 (137.795, 116.078) -> (137.795, 118.364)
  line L751 (139.065, 116.078) -> (137.795, 116.078)
  line L752 (139.065, 118.364) -> (139.065, 116.078)
  line L753 (137.795, 118.364) -> (139.065, 118.364)
  line L754 (140.335, 112.776) -> (140.335, 115.062)
  line L755 (140.335, 115.062) -> (141.5973, 115.062)
  line L756 (141.5973, 115.062) -> (141.5973, 112.776)
  line L757 (141.5973, 112.776) -> (140.335, 112.776)
  line L758 (142.875, 116.078) -> (142.875, 118.364)
  line L759 (142.875, 118.364) -> (144.145, 118.364)
  line L760 (144.145, 118.364) -> (144.145, 116.078)
  line L761 (144.145, 116.078) -> (142.875, 116.078)
  line L762 (145.415, 115.062) -> (146.6773, 115.062)
  line L763 (146.6773, 115.062) -> (146.6773, 112.776)
  line L764 (146.6773, 112.776) -> (145.415, 112.776)
  line L765 (145.415, 112.776) -> (145.415, 115.062)
  line L766 (127.635, 141.478) -> (127.635, 143.764)
  line L767 (127.635, 143.764) -> (128.905, 143.764)
  line L768 (128.905, 143.764) -> (128.905, 141.478)
  line L769 (128.905, 141.478) -> (127.635, 141.478)
  line L770 (130.175, 140.462) -> (131.4373, 140.462)
  line L771 (131.4373, 140.462) -> (131.4373, 138.176)
  line L772 (131.4373, 138.176) -> (130.175, 138.176)
  line L773 (130.175, 138.176) -> (130.175, 140.462)
  line L774 (133.985, 141.478) -> (132.715, 141.478)
  line L775 (133.985, 143.764) -> (133.985, 141.478)
  line L776 (132.715, 141.478) -> (132.715, 143.764)
  line L777 (132.715, 143.764) -> (133.985, 143.764)
  line L778 (135.255, 138.176) -> (135.255, 140.462)
  line L779 (136.5173, 138.176) -> (135.255, 138.176)
  line L780 (136.5173, 140.462) -> (136.5173, 138.176)
  line L781 (135.255, 140.462) -> (136.5173, 140.462)
  line L782 (137.795, 141.478) -> (137.795, 143.764)
  line L783 (139.065, 141.478) -> (137.795, 141.478)
  line L784 (139.065, 143.764) -> (139.065, 141.478)
  line L785 (137.795, 143.764) -> (139.065, 143.764)
  line L786 (140.335, 138.176) -> (140.335, 140.462)
  line L787 (140.335, 140.462) -> (141.5973, 140.462)
  line L788 (141.5973, 140.462) -> (141.5973, 138.176)
  line L789 (141.5973, 138.176) -> (140.335, 138.176)
  line L790 (142.875, 141.478) -> (142.875, 143.764)
  line L791 (142.875, 143.764) -> (144.145, 143.764)
  line L792 (144.145, 143.764) -> (144.145, 141.478)
  line L793 (144.145, 141.478) -> (142.875, 141.478)
  line L794 (145.415, 140.462) -> (146.6773, 140.462)
  line L795 (146.6773, 140.462) -> (146.6773, 138.176)
  line L796 (146.6773, 138.176) -> (145.415, 138.176)
  line L797 (145.415, 138.176) -> (145.415, 140.462)
  line L798 (127.635, 166.878) -> (127.635, 169.164)
  line L799 (127.635, 169.164) -> (128.905, 169.164)
  line L800 (128.905, 169.164) -> (128.905, 166.878)
  line L801 (128.905, 166.878) -> (127.635, 166.878)
  line L802 (130.175, 165.862) -> (131.4373, 165.862)
  line L803 (131.4373, 165.862) -> (131.4373, 163.576)
  line L804 (131.4373, 163.576) -> (130.175, 163.576)
  line L805 (130.175, 163.576) -> (130.175, 165.862)
  line L806 (133.985, 166.878) -> (132.715, 166.878)
  line L807 (133.985, 169.164) -> (133.985, 166.878)
  line L808 (132.715, 166.878) -> (132.715, 169.164)
  line L809 (132.715, 169.164) -> (133.985, 169.164)
  line L810 (135.255, 163.576) -> (135.255, 165.862)
  line L811 (136.5173, 163.576) -> (135.255, 163.576)
  line L812 (136.5173, 165.862) -> (136.5173, 163.576)
  line L813 (135.255, 165.862) -> (136.5173, 165.862)
  line L814 (137.795, 166.878) -> (137.795, 169.164)
  line L815 (139.065, 166.878) -> (137.795, 166.878)
  line L816 (139.065, 169.164) -> (139.065, 166.878)
  line L817 (137.795, 169.164) -> (139.065, 169.164)
  line L818 (140.335, 163.576) -> (140.335, 165.862)
  line L819 (140.335, 165.862) -> (141.5973, 165.862)
  line L820 (141.5973, 165.862) -> (141.5973, 163.576)
  line L821 (141.5973, 163.576) -> (140.335, 163.576)
  line L822 (142.875, 166.878) -> (142.875, 169.164)
  line L823 (142.875, 169.164) -> (144.145, 169.164)
  line L824 (144.145, 169.164) -> (144.145, 166.878)
  line L825 (144.145, 166.878) -> (142.875, 166.878)
  line L826 (145.415, 165.862) -> (146.6773, 165.862)
  line L827 (146.6773, 165.862) -> (146.6773, 163.576)
  line L828 (146.6773, 163.576) -> (145.415, 163.576)
  line L829 (145.415, 163.576) -> (145.415, 165.862)
  line L830 (127.635, 192.278) -> (127.635, 194.564)
  line L831 (127.635, 194.564) -> (128.905, 194.564)
  line L832 (128.905, 194.564) -> (128.905, 192.278)
  line L833 (128.905, 192.278) -> (127.635, 192.278)
  line L834 (130.175, 191.262) -> (131.4373, 191.262)
  line L835 (131.4373, 191.262) -> (131.4373, 188.976)
  line L836 (131.4373, 188.976) -> (130.175, 188.976)
  line L837 (130.175, 188.976) -> (130.175, 191.262)
  line L838 (133.985, 192.278) -> (132.715, 192.278)
  line L839 (133.985, 194.564) -> (133.985, 192.278)
  line L840 (132.715, 192.278) -> (132.715, 194.564)
  line L841 (132.715, 194.564) -> (133.985, 194.564)
  line L842 (135.255, 188.976) -> (135.255, 191.262)
  line L843 (136.5173, 188.976) -> (135.255, 188.976)
  line L844 (136.5173, 191.262) -> (136.5173, 188.976)
  line L845 (135.255, 191.262) -> (136.5173, 191.262)
  line L846 (137.795, 192.278) -> (137.795, 194.564)
  line L847 (139.065, 192.278) -> (137.795, 192.278)
  line L848 (139.065, 194.564) -> (139.065, 192.278)
  line L849 (137.795, 194.564) -> (139.065, 194.564)
  line L850 (140.335, 188.976) -> (140.335, 191.262)
  line L851 (140.335, 191.262) -> (141.5973, 191.262)
  line L852 (141.5973, 191.262) -> (141.5973, 188.976)
  line L853 (141.5973, 188.976) -> (140.335, 188.976)
  line L854 (142.875, 192.278) -> (142.875, 194.564)
  line L855 (142.875, 194.564) -> (144.145, 194.564)
  line L856 (144.145, 194.564) -> (144.145, 192.278)
  line L857 (144.145, 192.278) -> (142.875, 192.278)
  line L858 (145.415, 191.262) -> (146.6773, 191.262)
  line L859 (146.6773, 191.262) -> (146.6773, 188.976)
  line L860 (146.6773, 188.976) -> (145.415, 188.976)
  line L861 (145.415, 188.976) -> (145.415, 191.262)
  line L862 (0, 0) -> (17.78, 0) construction
  line L863 (17.78, 0) -> (17.78, 22.86) construction
  line L864 (17.78, 22.86) -> (0, 22.86) construction
  line L865 (0, 22.86) -> (0, 0) construction
  circle A0 centre (17.78, 22.86) radius 0.508
  line L866 (17.78, 22.86) -> (33.02, 22.86) construction
  line L867 (17.78, 22.86) -> (33.02, 22.86) construction
  circle A1 centre (33.02, 22.86) radius 0.508
  line L868 (25.4, 22.86) -> (25.4, 27.94) construction
  circle A2 centre (25.4, 27.94) radius 0.508
  circle A3 centre (43.18, 22.86) radius 0.508
  circle A4 centre (50.8, 27.94) radius 0.508
  circle A5 centre (58.42, 22.86) radius 0.508
  circle A6 centre (68.58, 22.86) radius 0.508
  circle A7 centre (76.2, 27.94) radius 0.508
  circle A8 centre (83.82, 22.86) radius 0.508
  circle A9 centre (93.98, 22.86) radius 0.508
  circle A10 centre (101.6, 27.94) radius 0.508
  circle A11 centre (109.22, 22.86) radius 0.508
  circle A12 centre (119.38, 22.86) radius 0.508
  circle A13 centre (127, 27.94) radius 0.508
  circle A14 centre (134.62, 22.86) radius 0.508
  circle A15 centre (144.78, 22.86) radius 0.508
  circle A16 centre (152.4, 27.94) radius 0.508
  circle A17 centre (160.02, 22.86) radius 0.508
  circle A18 centre (170.18, 22.86) radius 0.508
  circle A19 centre (177.8, 27.94) radius 0.508
  circle A20 centre (185.42, 22.86) radius 0.508
  circle A21 centre (195.58, 22.86) radius 0.508
  circle A22 centre (203.2, 27.94) radius 0.508
  circle A23 centre (210.82, 22.86) radius 0.508
  circle A24 centre (17.78, 48.26) radius 0.508
  circle A25 centre (25.4, 53.34) radius 0.508
  circle A26 centre (33.02, 48.26) radius 0.508
  circle A27 centre (43.18, 48.26) radius 0.508
  circle A28 centre (50.8, 53.34) radius 0.508
  circle A29 centre (58.42, 48.26) radius 0.508
  circle A30 centre (68.58, 48.26) radius 0.508
  circle A31 centre (76.2, 53.34) radius 0.508
  circle A32 centre (83.82, 48.26) radius 0.508
  circle A33 centre (93.98, 48.26) radius 0.508
  circle A34 centre (101.6, 53.34) radius 0.508
  circle A35 centre (109.22, 48.26) radius 0.508
  circle A36 centre (119.38, 48.26) radius 0.508
  circle A37 centre (127, 53.34) radius 0.508
  circle A38 centre (134.62, 48.26) radius 0.508
  circle A39 centre (144.78, 48.26) radius 0.508
  circle A40 centre (152.4, 53.34) radius 0.508
  circle A41 centre (160.02, 48.26) radius 0.508
  circle A42 centre (170.18, 48.26) radius 0.508
  circle A43 centre (177.8, 53.34) radius 0.508
  circle A44 centre (185.42, 48.26) radius 0.508
  circle A45 centre (195.58, 48.26) radius 0.508
  circle A46 centre (203.2, 53.34) radius 0.508
  circle A47 centre (210.82, 48.26) radius 0.508
  circle A48 centre (17.78, 73.66) radius 0.508
  circle A49 centre (25.4, 78.74) radius 0.508
  circle A50 centre (33.02, 73.66) radius 0.508
  circle A51 centre (43.18, 73.66) radius 0.508
  circle A52 centre (50.8, 78.74) radius 0.508
  circle A53 centre (58.42, 73.66) radius 0.508
  circle A54 centre (68.58, 73.66) radius 0.508
  circle A55 centre (76.2, 78.74) radius 0.508
  circle A56 centre (83.82, 73.66) radius 0.508
  circle A57 centre (93.98, 73.66) radius 0.508
  circle A58 centre (101.6, 78.74) radius 0.508
  circle A59 centre (109.22, 73.66) radius 0.508
  circle A60 centre (119.38, 73.66) radius 0.508
  circle A61 centre (127, 78.74) radius 0.508
  circle A62 centre (134.62, 73.66) radius 0.508
  circle A63 centre (144.78, 73.66) radius 0.508
  circle A64 centre (152.4, 78.74) radius 0.508
  circle A65 centre (160.02, 73.66) radius 0.508
  circle A66 centre (170.18, 73.66) radius 0.508
  circle A67 centre (177.8, 78.74) radius 0.508
  circle A68 centre (185.42, 73.66) radius 0.508
  circle A69 centre (195.58, 73.66) radius 0.508
  circle A70 centre (203.2, 78.74) radius 0.508
  circle A71 centre (210.82, 73.66) radius 0.508
  circle A72 centre (17.78, 99.06) radius 0.508
  circle A73 centre (25.4, 104.14) radius 0.508
  circle A74 centre (33.02, 99.06) radius 0.508
  circle A75 centre (43.18, 99.06) radius 0.508
  circle A76 centre (50.8, 104.14) radius 0.508
  circle A77 centre (58.42, 99.06) radius 0.508
  circle A78 centre (68.58, 99.06) radius 0.508
  circle A79 centre (76.2, 104.14) radius 0.508
  circle A80 centre (83.82, 99.06) radius 0.508
  circle A81 centre (93.98, 99.06) radius 0.508
  circle A82 centre (101.6, 104.14) radius 0.508
  circle A83 centre (109.22, 99.06) radius 0.508
  circle A84 centre (119.38, 99.06) radius 0.508
  circle A85 centre (127, 104.14) radius 0.508
  circle A86 centre (134.62, 99.06) radius 0.508
  circle A87 centre (144.78, 99.06) radius 0.508